hy-vfd v2 (Autodesk Fusion 360 design; units mm, degrees)
Autodesk Fusion 360 part; units mm, degrees
sketch "Sketch1" plane through (0, 0, 0) normal (0, 1, 0) x (1, 0, 0)
  line L0 (0, 0) -> (60, 0)
  line L1 (60, 0) -> (60, 82.3)
  line L2 (60, 82.3) -> (0, 82.3)
  line L3 (0, 82.3) -> (0, 0)
  line L4 (0, 82.3) -> (60, 0)
  line L5 (60, 82.3) -> (0, 0)
  line L6 (57.75, 79.65) -> (2.25, 79.65)
  line L7 (2.25, 79.65) -> (2.25, 2.65)
  line L8 (2.25, 2.65) -> (57.75, 2.65)
  line L9 (57.75, 2.65) -> (57.75, 79.65)
  line L10 (57.75, 79.65) -> (2.25, 2.65) construction
  line L11 (2.25, 79.65) -> (57.75, 2.65) construction
  point P0 (30, 41.15)
  dimension "d1" = 60
  dimension "d2" = 82.3
  dimension "d3" = 55.5
  dimension "d4" = 77
  constraint horizontal L0
  constraint vertical L1
  constraint horizontal L2
  constraint vertical L3
  constraint coincident L0.start L3.end
  constraint horizontal L6
  constraint perpendicular L6 L7
  constraint parallel L6 L8
  constraint parallel L7 L9
  constraint coincident L10 P0
  constraint coincident L11 P0
  constraint midpoint L5 P0
  measures "d1" distance of L0.start L0.end
  measures "d2" distance of L0.start L2.end
  measures "d3" distance of L7.end L8.end
  measures "d4" distance of L6.end L7.end
extrude "Extrude1" add sketch "Sketch1" along normal blind 16.7 contours L0 L4 L5 L7 L8 L9 | L3 L4 L5 L7 | L1 L4 L5 L9 | L2 L4 L5 L6 L7 L9 makes body 1
sketch "Sketch2" plane through (0, 16.7, 0) normal (0, 1, 0) x (-1, 0, 0)
  line L0 (-57.75, -79.65) -> (-57.75, -2.65)
  line L1 (-57.75, -2.65) -> (-2.25, -2.65)
  line L2 (-2.25, -2.65) -> (-2.25, -79.65)
  line L3 (-2.25, -79.65) -> (-57.75, -79.65)
  line L4 (0, -82.3) -> (0, 0)
  line L5 (0, 0) -> (-60, 0)
  line L6 (-60, 0) -> (-60, -82.3)
  line L7 (-60, -82.3) -> (0, -82.3)
  line L8 (-2.25, -79.65) -> (-30, -79.65)
  circle A0 centre (-30, -79.65) radius 13.5
  line L9 (0, -98.3) -> (-64, -98.3)
  line L10 (-64, -98.3) -> (-64, -82.3)
  line L11 (4, -82.3) -> (4, -98.3)
  line L12 (4, -98.3) -> (0, -98.3)
  line L13 (0, -82.3) -> (0, 0)
  line L14 (4, 0) -> (4, -82.3)
  line L15 (-64, -82.3) -> (-64, 0)
  line L16 (4, 0) -> (4, 4)
  line L17 (4, 4) -> (-60, 4)
  line L18 (-60, 4) -> (-64, 4)
  line L19 (-64, 4) -> (-64, 0)
  line L20 (-2.25, -2.65) -> (-30, -2.65)
  line L21 (-30, -32.65) -> (-44, -32.65)
  line L22 (-30, -2.65) -> (-15, -2.65)
  line L23 (-44, -32.65) -> (-15, -32.65)
  line L24 (-15, -32.65) -> (-15, -2.65)
  line L25 (-15, -2.65) -> (-44, -2.65)
  line L26 (-44, -2.65) -> (-44, -32.65)
  dimension "d7" = 4
  dimension "d19" = 14
  dimension "d20" = 15
  constraint coincident L4.end L5.start
  constraint coincident L2.end L3.start
  constraint midpoint L3 L8.end
  constraint coincident L8.end A0.centre
  constraint horizontal L9
  constraint vertical L10
  constraint vertical L11
  constraint horizontal L12
  constraint vertical L13
  constraint vertical L14
  constraint coincident L1.end L2.start
  constraint midpoint L1 L20.end
  constraint horizontal L23
  constraint vertical L24
  constraint horizontal L25
  constraint vertical L26
  measures "d7" distance of L6.end L10.end
  measures "d19" distance of L21.start L21.end
  measures "d20" distance of L20.end L22.end
extrude "Extrude2" add sketch "Sketch2" along normal blind 3 separate body contours L0 L1 L2 L3 L4 L5 L6 L7 L8 A0 L13 L20 L22 L25 | L3 L7 L8 A0 | L9 L10 L11 L12 L14 L15 L16 L17 L18 L19 makes body 2
sketch "Sketch3" plane through (0, 0, 0) normal (0, -1, 0) x (1, 0, 0)
  line L0 (57.75, -2.65) -> (57.75, -79.65)
  line L1 (57.75, -79.65) -> (2.25, -79.65)
  line L2 (2.25, -79.65) -> (2.25, -2.65)
  line L3 (2.25, -2.65) -> (57.75, -2.65)
  line L4 (0, 0) -> (0, -82.3)
  line L5 (0, -82.3) -> (60, -82.3)
  line L6 (60, -82.3) -> (60, 0)
  line L7 (60, 0) -> (0, 0)
  line L8 (0, 0) -> (60, 0)
  line L9 (60, 0) -> (60, -82.3)
  line L10 (60, -82.3) -> (0, -82.3)
  line L11 (0, -82.3) -> (0, 0)
  constraint horizontal L8
  constraint vertical L9
  constraint horizontal L10
  constraint vertical L11
  constraint coincident L5.end L6.start
  constraint coincident L4.start L7.end
extrude "Extrude3" add sketch "Sketch3" along normal blind 2 contours L0 L1 L2 L3 | L4 L5 L6 L7 L8 L9 L10 L11 bodies 1
sketch "Sketch4" plane through (0, 19.7, 0) normal (0, 1, 0) x (-1, 0, 0)
  arc A0 (-43.2374, -82.3) -> (-16.7626, -82.3) centre (-30, -79.65) ccw
  line L0 (-43.2374, -82.3) -> (-16.7626, -82.3)
  line L1 (-57.75, -2.65) -> (-2.25, -2.65)
  line L2 (-2.25, -2.65) -> (-2.25, -79.65)
  line L3 (-2.25, -79.65) -> (-57.75, -79.65)
  line L4 (-57.75, -79.65) -> (-57.75, -2.65)
  line L5 (4, -98.3) -> (4, 4)
  line L6 (4, 4) -> (-64, 4)
  line L7 (-64, 4) -> (-64, -98.3)
  line L8 (-64, -98.3) -> (4, -98.3)
  line L9 (-2.25, -79.65) -> (-57.75, -79.65)
  line L10 (-2.25, -79.65) -> (-30, -79.65)
  circle A1 centre (-30, -79.65) radius 13.5
  constraint coincident L2.end L3.start
  constraint coincident L3.end L4.start
  constraint coincident A0.centre L10.end
extrude "Extrude4" cut sketch "Sketch4" against normal blind 20 contours A0 L0 A1 | L0 L3 L9 L10 A1 | L3 L9 L10 A1 bodies 1 2
sketch "Sketch5" plane through (0, 19.7, 0) normal (0, 1, 0) x (-1, 0, 0)
  arc A0 (-43.5, -79.65) -> (-16.5, -79.65) centre (-30, -79.65) ccw
  line L0 (-43.5, -79.65) -> (-57.75, -79.65)
  line L1 (-57.75, -79.65) -> (-57.75, -2.65)
  line L2 (-57.75, -2.65) -> (-2.25, -2.65)
  line L3 (-2.25, -2.65) -> (-2.25, -79.65)
  line L4 (-2.25, -79.65) -> (-16.5, -79.65)
  line L5 (4, -98.3) -> (4, 4)
  line L6 (4, 4) -> (-64, 4)
  line L7 (-64, 4) -> (-64, -98.3)
  line L8 (-64, -98.3) -> (4, -98.3)
  line L9 (-16.5, -79.65) -> (-43.5, -79.65)
  circle A1 centre (-30, -79.65) radius 15
  line L10 (-43.5, -79.65) -> (-45, -79.65)
  line L11 (-16.5, -79.65) -> (-15, -79.65)
  constraint coincident A0.end L4.end
  constraint coincident A0.start L0.start
  constraint concentric A0 A1
  constraint coincident A1 L10.end
  constraint coincident L0 L10.end
  constraint coincident A1 L11.end
  constraint coincident L4 L11.end
extrude "Extrude5" add sketch "Sketch5" against normal blind 20 separate body contours A0 L0 L4 A1 L10 L11 makes body 3
sketch "Sketch6" plane through (0, -0.3, 0) normal (0, -1, 0) x (1, 0, 0)
  line L0 (45, -79.65) -> (43.5, -79.65)
  arc A0 (16.5, -79.65) -> (43.5, -79.65) centre (30, -79.65) ccw
  line L1 (16.5, -79.65) -> (15, -79.65)
  arc A1 (15, -79.65) -> (45, -79.65) centre (30, -79.65) ccw
sketch "Sketch7" plane through (0, 0, 0) normal (0, 1, 0) x (-1, 0, 0)
  arc A0 (-16.5, -79.65) -> (-43.5, -79.65) centre (-30, -79.65) ccw
  line L0 (-16.5, -79.65) -> (-2.25, -79.65)
  line L1 (-2.25, -79.65) -> (-2.25, -2.65)
  line L2 (-2.25, -2.65) -> (-57.75, -2.65)
  line L3 (-57.75, -2.65) -> (-57.75, -79.65)
  line L4 (-57.75, -79.65) -> (-43.5, -79.65)
  circle A1 centre (-30, -79.65) radius 13.5
  constraint concentric A0 A1
  constraint coincident A0.end A1
extrude "Extrude6" add sketch "Sketch7" against normal blind 2 separate body contours A0 A1 makes body 4
combine "Combine1" operation add target body 1 tool bodies 2
combine "Combine2" operation add target body 1 tool bodies 3
combine "Combine3" operation add target body 1 tool bodies 4
move_body "Move1" bodies 1 to x (-1, 0, 0) y (0, -1, 0) z (0, 0, 1) at (-8, -4, 0)
sketch "Sketch8" plane through (0, -23.7, 0) normal (0, -1, 0) x (1, 0, 0)
  line L0 (-4, -98.3) -> (-4, 4)
  line L1 (-4, 4) -> (-72, 4)
  line L2 (-72, 4) -> (-72, -98.3)
  line L3 (-72, -98.3) -> (-4, -98.3)
  line L4 (-51.5, -79.65) -> (-65.75, -79.65)
  line L5 (-65.75, -79.65) -> (-65.75, -2.65)
  line L6 (-65.75, -2.65) -> (-10.25, -2.65)
  line L7 (-10.25, -2.65) -> (-10.25, -79.65)
  line L8 (-10.25, -79.65) -> (-24.5, -79.65)
  arc A0 (-51.5, -79.65) -> (-24.5, -79.65) centre (-38, -79.65) ccw
  line L9 (-51.5, -79.65) -> (-24.5, -79.65)
  arc A1 (-51.5, -79.65) -> (-24.5, -79.65) centre (-38, -79.65) ccw
  arc A2 (-50.5, -79.65) -> (-25.5, -79.65) centre (-38, -79.65) ccw
  dimension "d32" = -1
  constraint coincident L4.start A0.start
  constraint coincident L8.end A0.end
extrude "Extrude7" cut 1 faces at (-23.9267, -3.7, -83.0097) along direction (0, -1, 0) blind 17 on bodies 1 bodies 1
extrude "Extrude8" add sketch "Sketch8" against normal blind 20 contours A0 L9 A1 A2 bodies 1
sketch "Sketch9" plane through (0, -4, 0) normal (0, -1, 0) x (1, 0, 0)
  line L0 (-25.5, -79.65) -> (-10.25, -79.65)
  line L1 (-10.25, -79.65) -> (-10.25, -2.65)
  line L2 (-10.25, -2.65) -> (-65.75, -2.65)
  line L3 (-65.75, -2.65) -> (-65.75, -79.65)
  line L4 (-65.75, -79.65) -> (-50.5, -79.65)
  arc A0 (-50.5, -79.65) -> (-25.5, -79.65) centre (-38, -79.65) ccw
  line L5 (-65.75, -2.65) -> (-38, -2.65)
  line L6 (-38, -2.65) -> (-38, -14.65)
  line L7 (-38, -14.65) -> (-25, -14.65)
  line L8 (-25, -14.65) -> (-25, -2.65)
  line L9 (-38, -14.65) -> (-51, -14.65)
  line L10 (-51, -14.65) -> (-51.0099, -2.65)
  dimension "d37" = 12
  dimension "d38" = 13
  dimension "d39" = 13
  constraint coincident L2.end L3.start
  constraint midpoint L2 L5.end
  constraint perpendicular L5 L6
  constraint perpendicular L1 L7
  constraint coincident L2 L8.end
  constraint perpendicular L2 L8
  constraint perpendicular L6 L9
  constraint coincident L2 L10.end
  measures "d37" distance of L5.end L6.end
  measures "d38" distance of L6.end L7.end
  measures "d39" distance of L6.end L9.end
extrude "Extrude9" cut sketch "Sketch9" against normal blind 19 contours L2 L6 L7 L8 | L2 L5 L6 L9 L10 bodies 1
